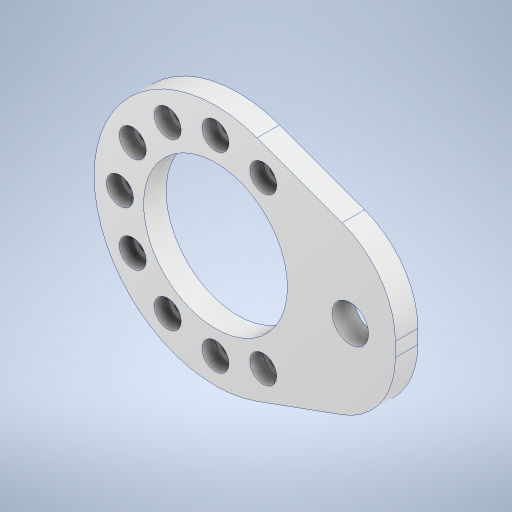
# Autodesk Inventor part: RP_Thigh-Base-Cover
Saved by Autodesk Inventor 2024.3 (Build 283343000, 343)
## iProperties
Created: 2024-10-20
Part Number: RP_Thigh-Base-Cover
Material: アルミニウム 6061
Document SubType Name: Modeling
Designer: 佐藤智貴
Density: 2.7 g/cm^3
Appearance: アルミニウム - フラット
Mass: 23.6781 g
Surface Area: 60.0306 cm^2
Volume: 8.76965 cm^3
Author: 佐藤智貴
Autodesk Inventor part; units mm, degrees
ref_plane "YZ Plane" through (0, 0, 0) normal (1, 0, 0) x (0, 1, 0)
ref_plane "XZ Plane" through (0, 0, 0) normal (0, 1, 0) x (-1, 0, 0)
ref_plane "作業平面1" through (0, 0, 14) normal (0, 0, 1) x (-0.9659, -0.2588, 0)
sketch "スケッチ14" plane through (0, 0, 0) normal (0, 0, 1) x (1, 0, 0)
  circle A0 centre (0, 0) radius 25
  circle A1 centre (30, 0) radius 4.05
  line L0 (0, 25) -> (40, 25)
  line L1 (40, 25) -> (40, -25)
  line L2 (40, -25) -> (0, -25)
  line L3 (0, -25) -> (0, 25)
  line L4 (0, -25) -> (40, -10.4412)
  line L5 (0, 25) -> (40, 10.4412)
  line L6 (0.5157, 26.4168) -> (40.5157, 11.858)
  line L7 (0.5157, -26.4168) -> (40.5157, -11.858)
  circle A2 centre (0, 0) radius 6.5
  circle A3 centre (0, 0) radius 28
  line L8 (1.5417, 29.2358) -> (41.5417, 14.677)
  line L9 (1.5417, -29.2358) -> (41.5417, -14.677)
  point P0 (8.5505, -23.4923)
  point P1 (40, -12.0456)
  point P2 (40, 12.0456)
  point P3 (8.5505, 23.4923)
  point P4 (40, 15.2382)
  point P5 (9.5766, 26.3114)
  point P6 (9.5766, -26.3114)
  point P7 (40, -15.2382)
  dimension "d111" = 50
  dimension "d112" = 8.1
  dimension "d113" = 30
  dimension "d114" = 40
  dimension "d115" = 50
  dimension "d116" = 25
  dimension "d119" = 25
  dimension "d126" = 20
  dimension "d127" = 20
  dimension "d144" = 13
  dimension "d207" = 3
  dimension "d208" = 3
  dimension "d209" = 3
  constraints: 20 end point, 6 parallel, 3 centre point, 2 coincident, 2 point on line, 1 horizontal, 1 perpendicular, 5 other
  measures "d112" diameter of A1
  measures "d113" distance of A3.centre A1.centre
  measures "d114" distance of L0.start L0.end
  measures "d115" distance between parallel lines of L2 L0
  measures "d116" distance from line of A3.centre L0
  measures "d119" distance from line of L0 A1.centre
  measures "d126" angle of L0 L5
  measures "d127" angle of L2 L4
  measures "d144" diameter of A2
  measures "d207" distance between parallel lines of L8 L6
  measures "d209" distance between parallel lines of L9 L7
extrude "押し出し9" add sketch "スケッチ14" along normal blind 5 contours L3 A2 A0 | L0 L6 A0 | A0 L2 A3 L0 | L5 A0 L4 L3 A2 | A0 L5 | L4 A0 | A0 L7 L2 | L6 A3 L5 A0 | L6 L0 A3 | L5 A3 A1 L4 A0 | L7 A3 L2 | A0 L4 A3 L7 | A3 L0 L8 L1 L6 | L6 L1 L5 A3 | A3 L8 L0 | L5 L1 L4 A3 A1 | A3 L4 L1 L7 | L7 L1 L9 L2 A3 | L2 L9 A3
sketch "スケッチ15" plane through (0, 0, 0) normal (0, 0, -1) x (-1, 0, 0)
  circle A0 centre (-30, 0) radius 4.05 projected
  circle A1 centre (-30, 0) radius 6.6
  point P0 (0, 0)
  dimension "d122" = 13.2
  constraints: 1 centre point, 1 coincident
  measures "d122" diameter of A1
extrude "押し出し10" cut sketch "スケッチ15" against normal blind 2
sketch "スケッチ16" plane through (0, 0, 5) normal (0, 0, 1) x (1, 0, 0)
  circle A0 centre (30, 0) radius 4.05 projected
  circle A1 centre (30, 0) radius 17
  arc A2 (8.5505, 23.4923) -> (8.5505, -23.4923) centre (0, 0) ccw projected
  circle A3 centre (0, 0) radius 25
  line L0 (40, -15.2382) -> (40, 15.2382) projected
  line L1 (40, 12.0456) -> (-0.2187, 26.6841)
  line L2 (40, -12.0456) -> (-2.6962, -27.5858)
  circle A4 centre (0, 0) radius 17.5
  line L3 (8.5505, 23.4923) -> (5.9854, 16.4446)
  line L4 (-17.5, 0) -> (-25, 0)
  line L5 (-2.7839, 19.6364) -> (32.5, 6.7941)
  line L6 (32.5, 6.7941) -> (32.5, -6.7941)
  line L7 (32.5, -6.7941) -> (-5.2613, -20.5381)
  line L8 (17.9474, 20.0721) -> (15.3823, 13.0244)
  point P0 (0, 25)
  point P1 (0, -25)
  dimension "d125" = 34
  dimension "d128" = 7.5
  dimension "d164" = 7.5
  dimension "d165" = 10
  constraints: 16 end point, 5 point on circle, 3 centre point, 3 coincident, 2 tangent, 1 parallel, 1 perpendicular, 2 other
  measures "d125" diameter of A1
  measures "d128" radial gap between concentric circles of A3 A4
  measures "d164" distance between parallel lines of L1 L5
  measures "d165" distance between parallel lines of L8 L3
extrude "押し出し11" add sketch "スケッチ16" along normal blind 10 contours L8 L5 L3 A3 | A3 L1 L8 | L3 A4 L4 A2
sketch "スケッチ17" plane through (0, 0, 5) normal (0, 0, 1) x (1, 0, 0)
  circle A0 centre (30, 0) radius 4.05 projected
  line L0 (0, 0) -> (30, 0)
  circle A1 centre (0, 0) radius 12.5
  line L1 (0, 0) -> (12.4415, 7.1831)
  point P0 (10.8253, 6.25)
  point P1 (0, 12.5)
  point P2 (-10.8253, 6.25)
  point P3 (-10.8253, -6.25)
  point P4 (0, -12.5)
  point P5 (10.8253, -6.25)
  dimension "d131" = 25
  dimension "d132" = 30
  dimension "d135" = 360
  constraints: 4 end point, 1 coincident, 1 horizontal, 1 point on line, 10 other
  measures "d132" angle of L0 L1
hole "穴5" at (10.8253, 6.25, 5) at (0, 12.5, 5) at (-10.8253, 6.25, 5) at (-10.8253, -6.25, 5) at (0, -12.5, 5) at (10.8253, -6.25, 5) direction (0, 0, -1) diameter 3.2 end through all
sketch "スケッチ18" plane through (0, 0, 5) normal (0, 0, 1) x (1, 0, 0)
  circle A0 centre (30, 0) radius 4.05 projected
  line L0 (0, 0) -> (30, 0)
  circle A1 centre (0, 0) radius 10.2
  point P0 (10.2, 0)
  point P1 (-5.1, 8.8335)
  point P2 (-5.1, -8.8335)
  dimension "d145" = 20.4
  dimension "d148" = 360
  constraints: 2 end point, 1 coincident, 1 horizontal, 1 horizontal alignment, 1 point on line, 6 other
hole "穴6" at (10.2, 0, 5) at (-5.1, 8.8335, 5) at (-5.1, -8.8335, 5) direction (0, 0, -1) diameter 4.2 end through all
sketch "スケッチ19" plane through (0, 0, 5) normal (0, 0, 1) x (1, 0, 0)
  circle A0 centre (0, 12.5) radius 1.6 projected
  circle A1 centre (0, 0) radius 12.5
  circle A2 centre (0, 12.5) radius 3
  circle A3 centre (-10.8253, 6.25) radius 3
  circle A4 centre (-10.8253, -6.25) radius 3
  circle A5 centre (0, -12.5) radius 3
  circle A6 centre (10.8253, -6.25) radius 3
  circle A7 centre (10.8253, 6.25) radius 3
  dimension "d157" = 6
  dimension "d160" = 360
  constraints: 6 centre point, 2 coincident, 1 vertical alignment, 15 other
  measures "d157" diameter of A2
extrude "押し出し12" cut sketch "スケッチ19" against normal blind 3 contours A0 A1 | A0 A1 A2 | A1 A0 | A0 A1 A2 | A3 A1 | A1 A3 | A7 A1 | A1 A7 | A4 A1 | A1 A4 | A6 A1 | A1 A6 | A5 A1 | A1 A5
sketch "スケッチ20" plane through (0, 0, 15) normal (0, 0, 1) x (1, 0, 0)
  line L0 (17.9474, 20.0721) -> (8.5505, 23.4923) projected
  line L1 (17.9474, 20.0721) -> (15.3823, 13.0244)
  line L2 (15.3823, 13.0244) -> (5.9854, 16.4446)
  line L3 (5.9854, 16.4446) -> (8.5505, 23.4923)
  line L4 (0, 0) -> (0, 30.7788)
  circle A0 centre (0, 0) radius 21.25
  circle A1 centre (0, 0) radius 25
  point P0 (11.9664, 18.2584)
  point P1 (0, 21.25)
  point P2 (-10.625, 18.403)
  point P3 (-18.403, 10.625)
  point P4 (-21.25, 0)
  point P5 (-18.403, -10.625)
  point P6 (-10.625, -18.403)
  point P7 (0, -21.25)
  point P8 (10.625, -18.403)
  point P9 (18.403, -10.625)
  point P10 (21.25, 0)
  point P11 (18.403, 10.625)
  point P12 (10.625, 18.403)
  dimension "d167" = 7.5
  dimension "d168" = 5
  dimension "d169" = 3.75
  dimension "d170" = 3.75
  dimension "d171" = 50
  dimension "d174" = 360
  constraints: 8 end point, 3 perpendicular, 2 coincident, 1 centre point, 1 point on line, 1 vertical, 1 vertical alignment, 15 other
  measures "d167" distance between parallel lines of L0 L2
  measures "d168" distance from line of L1 point (11.966, 18.258)
  measures "d169" distance from line of L2 point (11.966, 18.258)
  measures "d171" diameter of A1
hole "穴7" at (11.9664, 18.2584, 15) at (0, 21.25, 15) at (-10.625, 18.403, 15) at (-18.403, 10.625, 15) direction (0, 0, -1) diameter 2.459 end through all thread size "M3x0.5" class "6H" standard "ISO Metric profile"
sketch "スケッチ21" plane through (0, 0, 15) normal (0, 0, 1) x (1, 0, 0)
  circle A0 centre (0, 0) radius 25
  line L0 (40, -15.2382) -> (40, 15.2382) projected
  line L1 (40, 12.0456) -> (40, -12.0456)
  line L2 (8.5505, -23.4923) -> (40, -12.0456) projected
  line L3 (40, -12.0456) -> (8.5505, -23.4923)
  line L4 (40, 12.0456) -> (8.5505, 23.4923)
  line L5 (40, 0) -> (-25, 0)
  circle A1 centre (0, 0) radius 16
  circle A2 centre (30, 0) radius 4.05 projected
  circle A3 centre (30, 0) radius 4.05
  line L6 (9.2345, 25.3717) -> (42, 13.4461)
  line L7 (42, 13.4461) -> (42, -13.4461)
  line L8 (42, -13.4461) -> (9.2345, -25.3717)
  circle A4 centre (0, 0) radius 27
  line L9 (40, 15.2382) -> (40, -15.2382)
  point P0 (40, 14.174)
  point P1 (9.2345, 25.3717)
  point P2 (9.2345, -25.3717)
  point P3 (40, -14.174)
  dimension "d183" = 32
  dimension "d184" = 8.1
  dimension "d210" = 2
  dimension "d211" = 2
  constraints: 16 end point, 4 centre point, 3 coincident, 3 collinear, 2 point on circle, 2 tangent, 1 horizontal, 1 midpoint, 2 other
  measures "d183" diameter of A1
  measures "d184" diameter of A3
  measures "d210" distance between parallel lines of L4 L6
  measures "d211" radial gap between concentric circles of A0 A4
extrude "押し出し13" add sketch "スケッチ21" along normal blind 5 contours L5 A1 A0 | L5 A2 A4 L2 A0 | A0 L5 A1 | A0 L4 A4 A2 L5 | A0 L2 A4 L4 | A4 L6 L0 L4 | L4 L0 L5 A2 A4 | A4 A2 L5 L0 L2 | L2 L0 L8 A4
sketch "スケッチ22" plane through (0, 0, 20) normal (0, 0, 1) x (1, 0, 0)
  circle A0 centre (0, 21.25) radius 1.2295 projected
  circle A1 centre (0, 0) radius 21.25
  circle A2 centre (-10.625, 18.403) radius 1.2295 projected
  circle A3 centre (-18.403, 10.625) radius 1.2295 projected
  circle A4 centre (11.9664, 18.2584) radius 1.2295 projected
  line L0 (-17.5, 0) -> (-25, 0) projected
  line L1 (-25, 0) -> (40, 0)
  line L2 (40, -15.2382) -> (40, 15.2382) projected
  point P0 (40, -12.0456)
  point P1 (40, 12.0456)
  point P2 (0, -21.25)
  point P3 (-10.625, -18.403)
  point P4 (-18.403, -10.625)
  point P5 (11.9664, -18.2584)
  point P6 (-21.25, 0)
  point P7 (-18.403, 10.625)
  point P8 (-21.25, 0)
  point P9 (-18.403, -10.625)
  point P10 (-10.625, -18.403)
  point P11 (0, -21.25)
  point P12 (10.625, -18.403)
  point P13 (18.403, -10.625)
  point P14 (21.25, 0)
  point P15 (18.403, 10.625)
  point P16 (10.625, 18.403)
  point P17 (0, 21.25)
  dimension "d215" = 360
  constraints: 5 coincident, 4 symmetric about line, 2 end point, 2 point on circle, 1 centre point, 1 midpoint, 1 point on line, 13 other
hole "穴8" at (10.625, -18.403, 20) at (0, -21.25, 20) at (-10.625, -18.403, 20) at (-18.403, -10.625, 20) at (-18.403, 10.625, 20) at (-21.25, 0, 20) at (-10.625, 18.403, 20) at (0, 21.25, 20) at (10.625, 18.403, 20) direction (0, 0, -1) diameter 3.2 end through all
sketch "スケッチ23" plane through (0, 0, 0) normal (0, 0, -1) x (-1, 0, 0)
  line L0 (46.3543, -34.5724) -> (-56.544, -34.5724)
  line L1 (-56.544, -34.5724) -> (-56.544, 32.2069)
  line L2 (-56.544, 32.2069) -> (46.3543, 32.2069)
  line L3 (46.3543, 32.2069) -> (46.3543, -34.5724)
  point P0 (0, 0)
  constraints: 8 end point, 2 parallel, 1 horizontal, 1 perpendicular
extrude "押し出し14" cut sketch "スケッチ23" against normal blind 15
sketch "スケッチ24" plane through (0, 0, 20) normal (0, 0, 1) x (1, 0, 0)
  circle A0 centre (0, 21.25) radius 1.6 projected
  circle A1 centre (0, 21.25) radius 3
  circle A2 centre (-10.625, 18.403) radius 1.6 projected
  circle A3 centre (-10.625, 18.403) radius 3
  circle A4 centre (-18.403, 10.625) radius 1.6 projected
  circle A5 centre (-18.403, 10.625) radius 3
  line L0 (0, 0) -> (-8.2063, 0)
  circle A6 centre (0, -21.25) radius 3
  circle A7 centre (-10.625, -18.403) radius 3
  circle A8 centre (-18.403, -10.625) radius 3
  circle A9 centre (-21.25, -0.0076) radius 3
  circle A10 centre (0, 0) radius 21.25
  circle A11 centre (10.625, 18.403) radius 1.6 projected
  circle A12 centre (10.625, 18.403) radius 3
  circle A13 centre (10.625, -18.403) radius 1.6 projected
  circle A14 centre (10.625, -18.403) radius 3
  dimension "d198" = 6
  dimension "d199" = 6
  dimension "d200" = 6
  dimension "d203" = 6
  dimension "d217" = 6
  dimension "d218" = 6
  constraints: 10 centre point, 6 coincident, 3 symmetric about line, 2 end point, 2 point on circle, 1 horizontal, 3 other
  measures "d198" diameter of A1
  measures "d199" diameter of A3
  measures "d200" diameter of A5
  measures "d203" diameter of A9
  measures "d217" diameter of A14
  measures "d218" diameter of A12
extrude "押し出し15" cut sketch "スケッチ24" against normal blind 3 contours A0 A10 | A0 A10 A1 | A10 A0 | A0 A10 A1 | A10 A2 A3 | A3 A10 A2 | A12 A10 A11 | A10 A11 A12 | A10 A2 | A2 A10 | A10 A4 A5 | A5 A10 A4 | A14 A10 A13 | A10 A13 A14 | A10 A9 | A9 A10 | A10 A6 | A6 A10 | A10 A8 | A8 A10 | A10 A7 | A7 A10
fillet "フィレット10" radius 18 2 edges at (40, 14.174, 17.5) (40, -14.174, 17.5)
